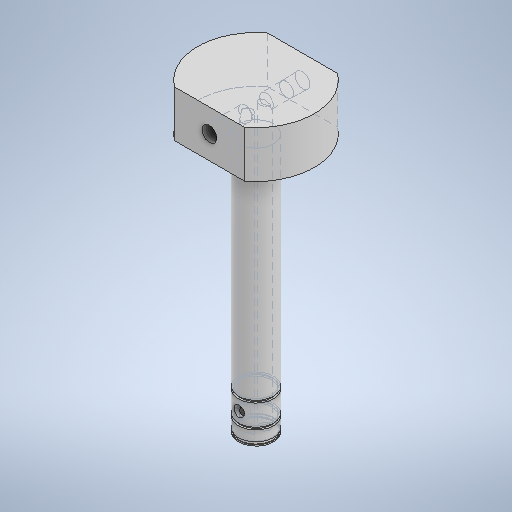
# Autodesk Inventor part: Passthrough Spindle
Saved by Autodesk Inventor 2025 (Build 290162000, 162)
## iProperties
Created: 2024-04-16
Part Number: Passthrough Spindle
Material: Generic
Document SubType Name: Modeling
Designer: cfang
Density: 1 g/cm^3
Appearance: Default
Author: cfang
Autodesk Inventor part; units mm, degrees
ref_plane "YZ Plane" through (0, 0, 0) normal (1, 0, 0) x (0, 1, 0)
ref_plane "XZ Plane" through (0, 0, 0) normal (0, 1, 0) x (-1, 0, 0)
ref_plane "XY Plane" through (0, 0, 0) normal (0, 0, 1) x (1, 0, 0)
sketch "Sketch1" plane through (0, 0, 0) normal (0, 1, 0) x (-1, 0, 0)
  circle A0 centre (0, 0) radius 7.5
  dimension "d0" = 15
  constraints: 1 centre point, 1 coincident
  measures "d0" diameter of A0
extrude "Extrusion1" add sketch "Sketch1" along normal blind 110.75
sketch "Sketch3" plane through (0, 110.75, 0) normal (0, 1, 0) x (1, 0, 0)
  circle A0 centre (0, 0) radius 7.5 projected
  circle A1 centre (0, 0) radius 25
  dimension "d12" = 50
  constraints: 1 centre point, 1 coincident
  measures "d12" diameter of A1
extrude "Extrusion2" add sketch "Sketch3" along normal blind 20 contours A0 | A1
sketch "Sketch5" plane through (0, 130.75, 0) normal (0, 1, 0) x (1, 0, 0)
  circle A0 centre (0, 0) radius 25 projected
  line L0 (15, 20) -> (-15, 20)
  line L1 (15, -20) -> (-15, -20)
  dimension "d24" = 20
  dimension "d25" = 20
  constraints: 4 end point, 4 point on circle, 2 horizontal alignment
  measures "d24" distance from line of L0 point (0, 0)
  measures "d25" distance from line of L1 point (0, 0)
extrude "Extrusion3" cut sketch "Sketch5" against normal through all contours L0 A0 | A0 L1
sketch "Sketch7" plane through (0, 0, 0) normal (0, -1, 0) x (1, 0, 0)
  point P0 (0, 0)
  point P1 (0, -3.75)
  point P2 (0, 3.75)
  dimension "d39" = 3.75
  dimension "d40" = 3.75
  measures "d39" distance of point (0, -3.75) point (0, 0)
  measures "d40" distance of point (0, 3.75) point (0, 0)
hole "Hole4" at (0, 0, -3.75) at (0, 0, 3.75) direction (0, 1, 0) diameter 4.5 depth 120.75 tip angle 118
sketch "Sketch6" plane through (15, 130.75, -20) normal (0, 0, -1) x (-1, 0, 0)
  line L0 (0, 0) -> (-10, 0) projected
  line L1 (0, -20) -> (-10, -20) projected
  line L2 (30, -20) -> (0, -20) projected
  point P0 (15, -130.75)
  point P1 (15, -10)
  dimension "d28" = 20
  dimension "d29" = 10
  measures "d28" distance between parallel lines of L0 L1
  measures "d29" distance from line of L2 point (15, -10)
hole "Hole3" at (0, 120.75, -20) direction (0, 0, 1) diameter 5.9436 depth 15.5 tip angle 118 taper from width 6.3893 to width 5.9591 over 6.8859 thread size "1/16" designation "1/16 - 27 NPT" standard "NPT"
sketch "Sketch8" plane through (-15, 130.75, 20) normal (0, 0, 1) x (1, 0, 0)
  line L0 (0, -20) -> (-10, -20) projected
  line L1 (0, 0) -> (-10, 0) projected
  point P0 (15, -130.75)
  point P1 (15, -10)
  dimension "d48" = 20
  dimension "d49" = 10
  measures "d48" distance between parallel lines of L0 L1
  measures "d49" distance from line of L0 point (15, -10)
hole "Hole5" at (0, 120.75, 20) direction (0, 0, -1) diameter 5.9436 depth 15.5 tip angle 118 taper from width 6.3651 to width 5.9936 over 5.9461 thread size "1/16" designation "1/16 - 27 NPT" standard "NPT for PVC Pipe and Fitting"
sketch "Sketch9" plane through (-15, 130.75, 20) normal (0, 0, 1) x (1, 0, 0)
  line L0 (22.5, -130.75) -> (7.5, -130.75) projected
  point P0 (15, -130.75)
  point P1 (15, -119.25)
  dimension "d59" = 11.5
  measures "d59" distance from line of L0 point (15, -119.25)
hole "Hole6" at (0, 11.5, 20) direction (0, 0, -1) diameter 4.5 depth 15.5 tip angle 118
sketch "Sketch11" plane through (0, 0, 0) normal (0, 0, 1) x (1, 0, 0)
  line L0 (7.5, 0) -> (7.5, 110.75) projected
  line L1 (7.5, 16) -> (6.7, 16)
  line L2 (6.7, 16) -> (6.7, 17)
  line L3 (6.7, 17) -> (7.5, 17)
  line L4 (7.5, 17) -> (7.5, 16)
  line L5 (0, 0) -> (0, 58.8907) construction
  line L6 (2.25, 120.75) -> (2.25, 0) construction
  line L7 (7.5, 0) -> (-7.5, 0) projected
  line L8 (7.5, 6) -> (6.7, 6)
  line L9 (6.7, 6) -> (6.7, 7)
  line L10 (6.7, 7) -> (7.5, 7)
  line L11 (7.5, 7) -> (7.5, 6)
  line L12 (7.5, 1.6) -> (7.15, 1.6)
  line L13 (7.15, 1.6) -> (7.15, 0.5)
  line L14 (7.15, 0.5) -> (7.5, 0.5)
  line L15 (7.5, 0.5) -> (7.5, 1.6)
  point P0 (7.5, 17)
  dimension "d78" = 0.8
  dimension "d79" = 1
  dimension "d80" = 16
  dimension "d81" = 0.8
  dimension "d82" = 1
  dimension "d83" = 6
  dimension "d84" = 0.35
  dimension "d85" = 1.1
  dimension "d86" = 0.5
  constraints: 26 end point, 7 parallel, 3 horizontal, 3 perpendicular, 3 point on line
  measures "d78" distance of L2.end L3.end
  measures "d79" distance of L1.end L2.end
  measures "d80" distance from line of L7 L1.end
  measures "d81" distance of L9.end L10.end
  measures "d82" distance of L8.end L9.end
  measures "d83" distance between parallel lines of L7 L8
  measures "d84" distance of L12.start L12.end
  measures "d85" distance of L12.end L13.end
  measures "d86" distance between parallel lines of L7 L14
revolve "Revolution1" cut sketch "Sketch11" angle 360 about axis through (0, 0, 0) along (0, 1, 0)
equation "\"d25\" = d24"
equation "\"d40\" = d39"
equation "\"d29\" = 0.5 * d28"
equation "\"d49\" = 0.5 * d48"
equation "\"d81\" = d78"
equation "\"d82\" = d79"
body "Solid1"
